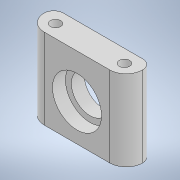
# Autodesk Inventor part: Крепление дифференциала
Saved by Autodesk Inventor 2020 (Build 240168000, 168)
## iProperties
Created: 2021-05-24
Part Number: Крепление дифференциала
Material: Типовые
Document SubType Name: Modeling
Designer: Антон
Density: 1 g/cm^3
Appearance: По умолчанию
Author: Антон
Autodesk Inventor part; units mm, degrees
ref_plane "YZ Plane" through (0, 0, 0) normal (1, 0, 0) x (0, 1, 0)
ref_plane "XZ Plane" through (0, 0, 0) normal (0, 1, 0) x (-1, 0, 0)
ref_plane "XY Plane" through (0, 0, 0) normal (0, 0, 1) x (1, 0, 0)
sketch "Эскиз1" plane through (0, 0, 0) normal (0, 0, 1) x (1, 0, 0)
  circle A0 centre (0, 0) radius 5.75
  circle A1 centre (0, 0) radius 9.55
  line L0 (9.55, 13.5) -> (-9.55, 13.5)
  line L1 (-9.55, 13.5) -> (-9.55, 0)
  line L2 (-9.55, 0) -> (9.55, 0)
  line L3 (9.55, 0) -> (9.55, 13.5)
  line L4 (9.55, 0) -> (-9.55, 0)
  line L5 (-9.55, 0) -> (-9.55, -11.3)
  line L6 (-9.55, -11.3) -> (9.55, -11.3)
  line L7 (9.55, -11.3) -> (9.55, 0)
  point P0 (9.55, 0)
  point P1 (0, 9.55)
  point P2 (-9.55, 0)
  point P3 (9.55, 0)
  point P4 (-9.55, 0)
  dimension "d0" = 11.5
  dimension "d1" = 19.1
  dimension "d64" = 11.3
  dimension "d85" = 13.5
  constraints: 16 end point, 4 parallel, 3 coincident, 2 centre point, 2 horizontal, 2 perpendicular, 1 midpoint, 1 tangent
  measures "d0" diameter of A0
  measures "d1" diameter of A1
  measures "d64" distance of L1.end L5.end
  measures "d85" distance of L2.end L0.start
extrude "Выдавливание1" add sketch "Эскиз1" along normal blind 8 contours L2 A1 A0 | A0 L2 A1 | L7 L6 L5 A1 | A1 L1 L0 L3
sketch "Эскиз15" plane through (0, 0, 8) normal (0, 0, 1) x (1, 0, 0)
  circle A0 centre (0, 0) radius 5.75 projected
  circle A1 centre (0, 0) radius 7.55
  dimension "d67" = 15.1
  constraints: 1 centre point, 1 coincident
  measures "d67" diameter of A1
extrude "Выдавливание9" cut sketch "Эскиз15" against normal blind 4
ref_plane "РабПлоскость6" through (0, -11.3, 0) normal (1, 0, 0) x (0, 0, -1)
sketch "Эскиз16" plane through (-9.55, -11.3, 0) normal (0, -1, 0) x (1, 0, 0)
  line L0 (0, 8) -> (19.1, 8) projected
  line L1 (19.1, 8) -> (24.7, 8)
  line L2 (24.7, 8) -> (24.7, 0)
  line L3 (24.7, 0) -> (19.1, 0)
  line L4 (19.1, 0) -> (19.1, 8)
  point P0 (9.55, 0)
  dimension "d70" = 5.6
  dimension "d71" = 8
  constraints: 8 end point, 2 parallel, 1 horizontal, 1 perpendicular
  measures "d70" distance of L2.end L3.end
  measures "d71" distance of L1.end L2.end
extrude "Выдавливание10" add sketch "Эскиз16" against normal up to surface (24.8 mm away)
sketch "Эскиз17" plane through (-9.55, 13.5, 0) normal (0, 1, 0) x (1, 0, 0)
  line L0 (24.7, 0) -> (24.7, -8) projected
  line L1 (24.7, -4) -> (20.15, -4)
  point P0 (9.55, 0)
  dimension "d82" = 4.55
  constraints: 2 end point, 1 coincident, 1 horizontal, 1 midpoint
  measures "d82" distance of L1.start L1.end
hole "Отверстие4" at (10.6, 13.5, 4) direction (0, -1, 0) diameter 3.2 end through all
fillet "Сопряжение5" radius 5.05 1 edges at (15.15, 1.1, 8)
fillet "Сопряжение5" radius 2.95 1 edges at (15.15, 1.1, 0)
mirror "Зеркальное отражение5" about plane through (0, -11.3, 0) normal (1, 0, 0) of "Сопряжение5", "Отверстие4", "Выдавливание10"
ref_plane "РабПлоскость7" through (0, -11.3, 0) normal (1, 0, 0) x (0, 0, -1)
